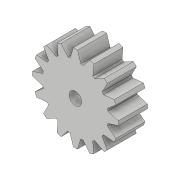
# Autodesk Inventor part: g
Saved by Autodesk Inventor 2019 (Build 230136000, 136)
## iProperties
Created: 2023-07-28
Part Number: g
Material: Generic
Document SubType Name: Modeling
Designer: ahmed
Density: 1 g/cm^3
Appearance: Default
Author: ahmed
## iProperties of the stored document g - Copy_3DPrint.ipt
Created: 2023-08-01
Part Number: g - Copy_3DPrint
Material: Generic
Document SubType Name: Modeling
Designer: ahmed
Density: 1 g/cm^3
Appearance: Default
Author: ahmed
Autodesk Inventor part; units mm, degrees
ref_plane "YZ Plane" through (0, 0, 0) normal (1, 0, 0) x (0, 1, 0)
ref_plane "XZ Plane" through (0, 0, 0) normal (0, 1, 0) x (-1, 0, 0)
ref_plane "XY Plane" through (0, 0, 0) normal (0, 0, 1) x (1, 0, 0)
sketch "Sketch3" plane through (0, 0, 0) normal (0, 0, 1) x (1, 0, 0)
  arc A0 (0.7179, 14.7325) -> (-0.7179, 14.7325) centre (0, 0) ccw
  circle A1 centre (0, 0) radius 2.15
  line L0 (0.7179, 14.7325) -> (1.8472, 11.1881)
  line L1 (-0.7179, 14.7325) -> (-1.8013, 11.1738)
  arc A2 (-4.9746, 13.8858) -> (-6.3011, 13.3363) centre (0, 0) ccw
  line L2 (-4.9746, 13.8858) -> (-2.5749, 11.0433)
  line L3 (-6.3011, 13.3363) -> (-5.9402, 9.6339)
  arc A3 (-9.9098, 10.9251) -> (-10.9251, 9.9098) centre (0, 0) ccw
  line L4 (-9.9098, 10.9251) -> (-6.605, 9.2173)
  line L5 (-10.9251, 9.9098) -> (-9.1747, 6.6274)
  arc A4 (-13.3363, 6.3011) -> (-13.8858, 4.9746) centre (0, 0) ccw
  line L6 (-13.3363, 6.3011) -> (-9.6295, 5.9881)
  line L7 (-13.8858, 4.9746) -> (-11.0125, 2.6119)
  arc A5 (-14.7325, 0.7179) -> (-14.7325, -0.7179) centre (0, 0) ccw
  line L8 (-14.7325, 0.7179) -> (-11.1881, 1.8472)
  line L9 (-14.7325, -0.7179) -> (-11.1738, -1.8013)
  arc A6 (-13.8858, -4.9746) -> (-13.3363, -6.3011) centre (0, 0) ccw
  line L10 (-13.8858, -4.9746) -> (-11.0433, -2.5749)
  line L11 (-13.3363, -6.3011) -> (-9.6339, -5.9402)
  arc A7 (-10.9251, -9.9098) -> (-9.9098, -10.9251) centre (0, 0) ccw
  line L12 (-10.9251, -9.9098) -> (-9.2173, -6.605)
  line L13 (-9.9098, -10.9251) -> (-6.6274, -9.1747)
  arc A8 (-6.3011, -13.3363) -> (-4.9746, -13.8858) centre (0, 0) ccw
  line L14 (-6.3011, -13.3363) -> (-5.9881, -9.6295)
  line L15 (-4.9746, -13.8858) -> (-2.6119, -11.0125)
  arc A9 (-0.7179, -14.7325) -> (0.7179, -14.7325) centre (0, 0) ccw
  line L16 (-0.7179, -14.7325) -> (-1.8472, -11.1881)
  line L17 (0.7179, -14.7325) -> (1.8013, -11.1738)
  arc A10 (4.9746, -13.8858) -> (6.3011, -13.3363) centre (0, 0) ccw
  line L18 (4.9746, -13.8858) -> (2.5749, -11.0433)
  line L19 (6.3011, -13.3363) -> (5.9402, -9.6339)
  arc A11 (9.9098, -10.9251) -> (10.9251, -9.9098) centre (0, 0) ccw
  line L20 (9.9098, -10.9251) -> (6.605, -9.2173)
  line L21 (10.9251, -9.9098) -> (9.1747, -6.6274)
  arc A12 (13.3363, -6.3011) -> (13.8858, -4.9746) centre (0, 0) ccw
  line L22 (13.3363, -6.3011) -> (9.6295, -5.9881)
  line L23 (13.8858, -4.9746) -> (11.0125, -2.6119)
  arc A13 (14.7325, -0.7179) -> (14.7325, 0.7179) centre (0, 0) ccw
  line L24 (14.7325, -0.7179) -> (11.1881, -1.8472)
  line L25 (14.7325, 0.7179) -> (11.1738, 1.8013)
  arc A14 (13.8858, 4.9746) -> (13.3363, 6.3011) centre (0, 0) ccw
  line L26 (13.8858, 4.9746) -> (11.0433, 2.5749)
  line L27 (13.3363, 6.3011) -> (9.6339, 5.9402)
  arc A15 (10.9251, 9.9098) -> (9.9098, 10.9251) centre (0, 0) ccw
  line L28 (10.9251, 9.9098) -> (9.2173, 6.605)
  line L29 (9.9098, 10.9251) -> (6.6274, 9.1747)
  arc A16 (6.3011, 13.3363) -> (4.9746, 13.8858) centre (0, 0) ccw
  line L30 (6.3011, 13.3363) -> (5.9881, 9.6295)
  line L31 (4.9746, 13.8858) -> (2.6119, 11.0125)
  arc A17 (-1.7943, 11.1967) -> (-2.5749, 11.0433) centre (0, 0) ccw
  arc A18 (2.6271, 11.031) -> (1.8472, 11.1881) centre (0, 0) ccw
  arc A19 (6.6485, 9.186) -> (5.9881, 9.6295) centre (0, 0) ccw
  arc A20 (9.6577, 5.9425) -> (9.2173, 6.605) centre (0, 0) ccw
  arc A21 (11.1967, 1.7943) -> (11.0433, 2.5749) centre (0, 0) ccw
  arc A22 (11.031, -2.6271) -> (11.1881, -1.8472) centre (0, 0) ccw
  arc A23 (9.186, -6.6485) -> (9.6295, -5.9881) centre (0, 0) ccw
  arc A24 (5.9425, -9.6577) -> (6.605, -9.2173) centre (0, 0) ccw
  arc A25 (1.7943, -11.1967) -> (2.5749, -11.0433) centre (0, 0) ccw
  arc A26 (-2.6271, -11.031) -> (-1.8472, -11.1881) centre (0, 0) ccw
  arc A27 (-6.6485, -9.186) -> (-5.9881, -9.6295) centre (0, 0) ccw
  arc A28 (-9.6577, -5.9425) -> (-9.2173, -6.605) centre (0, 0) ccw
  arc A29 (-11.1967, -1.7943) -> (-11.0433, -2.5749) centre (0, 0) ccw
  arc A30 (-11.031, 2.6271) -> (-11.1881, 1.8472) centre (0, 0) ccw
  arc A31 (-5.9425, 9.6577) -> (-6.605, 9.2173) centre (0, 0) ccw
  arc A32 (-9.186, 6.6485) -> (-9.6295, 5.9881) centre (0, 0) ccw
  point P0 (1.7935, 11.3568)
  point P1 (-2.6891, 11.1786)
  point P2 (-6.7623, 9.2986)
  point P3 (-9.806, 6.003)
  point P4 (-11.3568, 1.7935)
  point P5 (-11.1786, -2.6891)
  point P6 (-9.2986, -6.7623)
  point P7 (-6.003, -9.806)
  point P8 (-1.7935, -11.3568)
  point P9 (2.6891, -11.1786)
  point P10 (6.7623, -9.2986)
  point P11 (9.806, -6.003)
  point P12 (11.3568, -1.7935)
  point P13 (11.1786, 2.6891)
  point P14 (9.2986, 6.7623)
  point P15 (6.003, 9.806)
  dimension "d13" = 29.5
  dimension "d14" = 4.3
  dimension "d17" = 3.72
  dimension "d18" = 3.72
  dimension "d21" = 360
  constraints: 64 end point, 64 point on circle, 33 centre point, 16 point on line, 3 coincident, 145 other
  measures "d13" diameter of A0
  measures "d14" diameter of A1
  measures "d17" distance of L0.start L0.end
  measures "d18" distance of L1.start L1.end
extrude "Extrusion2" add sketch "Sketch3" along normal blind 10
body "Solid2"
